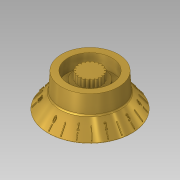
# Autodesk Inventor part: Knob
Saved by Autodesk Inventor 2016 (Build 200138000, 138)
## iProperties
Created: 2018-09-08
Part Number: Knob
Material: Generic
Document SubType Name: Modeling
Designer: Pedro Mendonça
Density: 1 g/cm^3
Appearance: Gold - Metal(1)
Author: Pedro Mendonça
Autodesk Inventor part; units mm, degrees
ref_plane "YZ Plane" through (0, 0, 0) normal (1, 0, 0) x (0, 1, 0)
ref_plane "XZ Plane" through (0, 0, 0) normal (0, 1, 0) x (-1, 0, 0)
sketch "Sketch1" plane through (0, 0, 0) normal (1, 0, 0) x (0, 1, 0)
  line L0 (0, 0) -> (0, 12.45)
  line L1 (0, 12.45) -> (8.7, 12.45)
  line L2 (8.7, 12.45) -> (9.2, 4.8665)
  line L3 (0, 0) -> (13.15, 0)
  line L4 (13.15, 0) -> (9.2, 4.8665)
  line L5 (0, -2.49) -> (0, 14.94) projected
  dimension "d5" = 12.45
  dimension "d6" = 8.7
  dimension "d7" = 7.6
  dimension "d8" = 13.15
  dimension "d10" = 9.2
  constraints: 10 end point, 1 horizontal, 1 perpendicular, 1 vertical
  measures "d5" distance of L0.start L0.end
  measures "d6" distance of L0.end L1.end
  measures "d7" distance of L1.end L2.end
  measures "d8" distance of L0.start L3.end
  measures "d10" distance from line of L2.end L0
revolve "Revolution1" add sketch "Sketch1" angle 360 about axis through (0, 0, -10) along (0, 0, 1)
sketch "Sketch2" plane through (0, 0, 0) normal (1, 0, 0) x (0, 1, 0)
  line L0 (-11.15, 0) -> (-7.2104, 4.8749)
  line L1 (-7.2173, 4.8665) -> (-6.8225, 10.8535)
  line L2 (-6.8225, 10.8535) -> (-4.8225, 10.8535)
  line L3 (-4.8225, 10.8535) -> (-4.8225, 0)
  line L4 (-11.15, 0) -> (-4.8225, 0)
  line L5 (-13.15, 0) -> (13.15, 0) projected
  line L6 (-11.15, 0) -> (-7.2173, 4.8665)
  line L7 (-6.8225, 10.8535) -> (-4.8225, 10.8535)
  line L8 (-4.8225, 0) -> (-11.15, 0)
  line L9 (0, -2.49) -> (0, 14.94) projected
  point P0 (0, 0)
  dimension "d14" = 6
  dimension "d15" = 2
  constraints: 16 end point, 2 horizontal, 2 parallel, 1 collinear
  measures "d14" distance of L1.start L1.end
  measures "d15" distance of L1.end L2.end
revolve "Revolution2" cut sketch "Sketch2" angle 360 about axis through (0, 0, -10) along (0, 0, 1)
sketch "Sketch3" plane through (0, 0, 0) normal (0, 0, -1) x (-1, 0, 0)
  circle A0 centre (0, 0) radius 3.125
  dimension "d17" = 6.25
  constraints: 1 centre point, 1 coincident
  measures "d17" diameter of A0
extrude "Extrusion1" cut sketch "Sketch3" against normal blind 8
sketch "Sketch4" plane through (0, 0, 0) normal (0, 0, -1) x (-1, 0, 0)
  circle A0 centre (0, 0) radius 3.125 projected
  circle A1 centre (0, -3.125) radius 0.485
  circle A2 centre (0.9657, -2.9721) radius 0.485
  circle A3 centre (1.8368, -2.5282) radius 0.485
  circle A4 centre (2.5282, -1.8368) radius 0.485
  circle A5 centre (2.9721, -0.9657) radius 0.485
  circle A6 centre (3.125, 0) radius 0.485
  circle A7 centre (2.9721, 0.9657) radius 0.485
  circle A8 centre (2.5282, 1.8368) radius 0.485
  circle A9 centre (1.8368, 2.5282) radius 0.485
  circle A10 centre (0.9657, 2.9721) radius 0.485
  circle A11 centre (0, 3.125) radius 0.485
  circle A12 centre (-0.9657, 2.9721) radius 0.485
  circle A13 centre (-1.8368, 2.5282) radius 0.485
  circle A14 centre (-2.5282, 1.8368) radius 0.485
  circle A15 centre (-2.9721, 0.9657) radius 0.485
  circle A16 centre (-3.125, 0) radius 0.485
  circle A17 centre (-2.9721, -0.9657) radius 0.485
  circle A18 centre (-2.5282, -1.8368) radius 0.485
  circle A19 centre (-1.8368, -2.5282) radius 0.485
  circle A20 centre (-0.9657, -2.9721) radius 0.485
  dimension "d20" = 0.97
  dimension "d23" = 360
  constraints: 20 centre point, 1 vertical alignment, 42 other
  measures "d20" diameter of A1
extrude "Extrusion2" cut sketch "Sketch4" against normal blind 8 contours A0 A6 | A0 A6 | A7 A0 | A0 A7 | A5 A0 | A0 A5 | A8 A0 | A0 A8 | A4 A0 | A0 A4 | A9 A0 | A0 A9 | A3 A0 | A0 A3 | A10 A0 | A0 A10 | A2 A0 | A0 A2 | A11 A0 | A0 A11 | A1 A0 | A0 A1 | A12 A0 | A0 A12 | A20 A0 | A0 A20 | A13 A0 | A0 A13 | A19 A0 | A0 A19 | A14 A0 | A0 A14 | A18 A0 | A0 A18 | A15 A0 | A0 A15 | A17 A0 | A0 A17 | A16 A0 | A0 A16
fillet "Fillet1" radius 1 1 edges at (0, -9.2, 4.8665)
fillet "Fillet3" radius 0.1 1 edges at (0, -13.15, 0)
sketch "Sketch7" plane through (0, 0, 12.45) normal (0, 0, 1) x (1, 0, 0)
  circle A0 centre (0, 0) radius 10
  dimension "d95" = 20
  constraints: 1 centre point, 1 coincident
  measures "d95" diameter of A0
extrude "Extrusion4" cut sketch "Sketch7" against normal blind 2
sketch "Sketch8" plane through (0, 0, 0) normal (0, 0, -1) x (-1, 0, 0)
  circle A0 centre (0, 0) radius 4.8225
  constraints: 1 centre point, 1 coincident
extrude "Extrusion5" cut sketch "Sketch8" against normal blind 2.5
sketch "Sketch9" plane through (0, 0, 10.45) normal (0, 0, 1) x (1, 0, 0)
  circle A0 centre (0, 0) radius 4.8225 projected
  arc A1 (-1.4235, 2.7819) -> (-2.2059, 2.2135) centre (-1.8368, 2.5282) ccw projected
  arc A2 (-0.4942, 3.0857) -> (-1.4139, 2.7868) centre (-0.9657, 2.9721) ccw projected
  arc A3 (0.4835, 3.0874) -> (-0.4835, 3.0874) centre (0, 3.125) ccw projected
  arc A4 (1.4139, 2.7868) -> (0.4942, 3.0857) centre (0.9657, 2.9721) ccw projected
  arc A5 (2.2059, 2.2135) -> (1.4235, 2.7819) centre (1.8368, 2.5282) ccw projected
  arc A6 (2.7819, 1.4235) -> (2.2135, 2.2059) centre (2.5282, 1.8368) ccw projected
  arc A7 (3.0857, 0.4942) -> (2.7868, 1.4139) centre (2.9721, 0.9657) ccw projected
  arc A8 (3.0874, -0.4835) -> (3.0874, 0.4835) centre (3.125, 0) ccw projected
  arc A9 (2.7868, -1.4139) -> (3.0857, -0.4942) centre (2.9721, -0.9657) ccw projected
  arc A10 (2.2135, -2.2059) -> (2.7819, -1.4235) centre (2.5282, -1.8368) ccw projected
  arc A11 (1.4235, -2.7819) -> (2.2059, -2.2135) centre (1.8368, -2.5282) ccw projected
  arc A12 (0.4942, -3.0857) -> (1.4139, -2.7868) centre (0.9657, -2.9721) ccw projected
  arc A13 (-0.4835, -3.0874) -> (0.4835, -3.0874) centre (0, -3.125) ccw projected
  arc A14 (-1.4139, -2.7868) -> (-0.4942, -3.0857) centre (-0.9657, -2.9721) ccw projected
  arc A15 (-2.2059, -2.2135) -> (-1.4235, -2.7819) centre (-1.8368, -2.5282) ccw projected
  arc A16 (-2.7819, -1.4235) -> (-2.2135, -2.2059) centre (-2.5282, -1.8368) ccw projected
  arc A17 (-3.0857, -0.4942) -> (-2.7868, -1.4139) centre (-2.9721, -0.9657) ccw projected
  arc A18 (-3.0874, 0.4835) -> (-3.0874, -0.4835) centre (-3.125, 0) ccw projected
  arc A19 (-2.7868, 1.4139) -> (-3.0857, 0.4942) centre (-2.9721, 0.9657) ccw projected
  arc A20 (-2.2135, 2.2059) -> (-2.7819, 1.4235) centre (-2.5282, 1.8368) ccw projected
  arc A21 (3.0857, -0.4942) -> (3.0874, -0.4835) centre (0, 0) ccw
  arc A22 (3.0874, 0.4835) -> (3.0857, 0.4942) centre (0, 0) ccw
  arc A23 (2.7868, 1.4139) -> (2.7819, 1.4235) centre (0, 0) ccw
  arc A24 (2.2135, 2.2059) -> (2.2059, 2.2135) centre (0, 0) ccw
  arc A25 (1.4235, 2.7819) -> (1.4139, 2.7868) centre (0, 0) ccw
  arc A26 (0.4942, 3.0857) -> (0.4835, 3.0874) centre (0, 0) ccw
  arc A27 (-0.4835, 3.0874) -> (-0.4942, 3.0857) centre (0, 0) ccw
  arc A28 (-1.4139, 2.7868) -> (-1.4235, 2.7819) centre (0, 0) ccw
  arc A29 (-2.2059, 2.2135) -> (-2.2135, 2.2059) centre (0, 0) ccw
  arc A30 (-2.7819, 1.4235) -> (-2.7868, 1.4139) centre (0, 0) ccw
  arc A31 (-3.0857, 0.4942) -> (-3.0874, 0.4835) centre (0, 0) ccw
  arc A32 (-3.0874, -0.4835) -> (-3.0857, -0.4942) centre (0, 0) ccw
  arc A33 (-2.7868, -1.4139) -> (-2.7819, -1.4235) centre (0, 0) ccw
  arc A34 (-2.2135, -2.2059) -> (-2.2059, -2.2135) centre (0, 0) ccw
  arc A35 (-1.4235, -2.7819) -> (-1.4139, -2.7868) centre (0, 0) ccw
  arc A36 (-0.4942, -3.0857) -> (-0.4835, -3.0874) centre (0, 0) ccw
  arc A37 (0.4835, -3.0874) -> (0.4942, -3.0857) centre (0, 0) ccw
  arc A38 (1.4139, -2.7868) -> (1.4235, -2.7819) centre (0, 0) ccw
  arc A39 (2.2059, -2.2135) -> (2.2135, -2.2059) centre (0, 0) ccw
  arc A40 (2.7819, -1.4235) -> (2.7868, -1.4139) centre (0, 0) ccw
  constraints: 80 point on circle, 20 centre point, 1 coincident
extrude "Extrusion6" cut sketch "Sketch9" against normal blind 2.3
ref_plane "Work Plane2" through (0, 0, 6.15) normal (0, 0, 1) x (1, 0, 0)
sketch "Sketch11" plane through (0, 0, 6.15) normal (0, 0, 1) x (1, 0, 0)
  circle A0 centre (0, 0) radius 7.75
  circle A1 centre (0, 0) radius 4.8212
  dimension "d106" = 15.5
  constraints: 2 centre point, 2 coincident
  measures "d106" diameter of A0
extrude "Extrusion9" add sketch "Sketch11" against normal blind 1
ref_plane "Work Plane3" through (0, 0, 20) normal (0, 0, 1) x (1, 0, 0)
sketch "Sketch12" plane through (0, 0, 20) normal (0, 0, 1) x (1, 0, 0)
  line L0 (12.8, -0.1) -> (11.8, -0.1)
  line L1 (11.8, -0.1) -> (11.8, 0.1)
  line L2 (11.8, 0.1) -> (12.8, 0.1)
  line L3 (12.8, 0.1) -> (12.8, -0.1)
  line L4 (12.8, -0.1) -> (11.8, 0.1) construction
  line L5 (11.8, -0.1) -> (12.8, 0.1) construction
  line L6 (10.4579, 2.6987) -> (12.3897, 3.2163)
  line L7 (12.3897, 3.2163) -> (12.338, 3.4095)
  line L8 (12.338, 3.4095) -> (10.4061, 2.8918)
  line L9 (10.4061, 2.8918) -> (10.4579, 2.6987)
  line L10 (10.9468, 6.6346) -> (10.0957, 6.1096)
  line L11 (10.0957, 6.1096) -> (9.9907, 6.2798)
  line L12 (9.9907, 6.2798) -> (10.8418, 6.8048)
  line L13 (10.8418, 6.8048) -> (10.9468, 6.6346)
  line L14 (10.9468, 6.6346) -> (9.9907, 6.2798) construction
  line L15 (10.0957, 6.1096) -> (10.8418, 6.8048) construction
  line L16 (7.4841, 7.787) -> (8.8566, 9.2418)
  line L17 (8.8566, 9.2418) -> (8.7112, 9.379)
  line L18 (8.7112, 9.379) -> (7.3387, 7.9243)
  line L19 (7.3387, 7.9243) -> (7.4841, 7.787)
  line L20 (5.834, 11.3936) -> (5.3852, 10.5)
  line L21 (5.3852, 10.5) -> (5.2065, 10.5897)
  line L22 (5.2065, 10.5897) -> (5.6553, 11.4834)
  line L23 (5.6553, 11.4834) -> (5.834, 11.3936)
  line L24 (5.834, 11.3936) -> (5.2065, 10.5897) construction
  line L25 (5.3852, 10.5) -> (5.6553, 11.4834) construction
  line L26 (2.2819, 10.5567) -> (2.6863, 12.5153)
  line L27 (2.6863, 12.5153) -> (2.4905, 12.5558)
  line L28 (2.4905, 12.5558) -> (2.086, 10.5971)
  line L29 (2.086, 10.5971) -> (2.2819, 10.5567)
  line L30 (-1.016, 12.76) -> (-0.9288, 11.7638)
  line L31 (-0.9288, 11.7638) -> (-1.1281, 11.7464)
  line L32 (-1.1281, 11.7464) -> (-1.2152, 12.7426)
  line L33 (-1.2152, 12.7426) -> (-1.016, 12.76)
  line L34 (-1.016, 12.76) -> (-1.1281, 11.7464) construction
  line L35 (-0.9288, 11.7638) -> (-1.2152, 12.7426) construction
  line L36 (-3.5998, 10.1829) -> (-4.2839, 12.0623)
  line L37 (-4.2839, 12.0623) -> (-4.4718, 11.9939)
  line L38 (-4.4718, 11.9939) -> (-3.7878, 10.1145)
  line L39 (-3.7878, 10.1145) -> (-3.5998, 10.1829)
  line L40 (-7.5634, 10.3269) -> (-6.9663, 9.5248)
  line L41 (-6.9663, 9.5248) -> (-7.1267, 9.4053)
  line L42 (-7.1267, 9.4053) -> (-7.7238, 10.2075)
  line L43 (-7.7238, 10.2075) -> (-7.5634, 10.3269)
  line L44 (-7.5634, 10.3269) -> (-7.1267, 9.4053) construction
  line L45 (-6.9663, 9.5248) -> (-7.7238, 10.2075) construction
  line L46 (-8.4097, 6.777) -> (-9.9785, 8.0175)
  line L47 (-9.9785, 8.0175) -> (-10.1025, 7.8606)
  line L48 (-10.1025, 7.8606) -> (-8.5337, 6.6201)
  line L49 (-8.5337, 6.6201) -> (-8.4097, 6.777)
  line L50 (-11.8587, 4.8188) -> (-10.9294, 4.4496)
  line L51 (-10.9294, 4.4496) -> (-11.0032, 4.2637)
  line L52 (-11.0032, 4.2637) -> (-11.9326, 4.6329)
  line L53 (-11.9326, 4.6329) -> (-11.8587, 4.8188)
  line L54 (-11.8587, 4.8188) -> (-11.0032, 4.2637) construction
  line L55 (-10.9294, 4.4496) -> (-11.9326, 4.6329) construction
  line L56 (-10.7154, 1.3531) -> (-12.7018, 1.5853)
  line L57 (-12.7018, 1.5853) -> (-12.7251, 1.3867)
  line L58 (-12.7251, 1.3867) -> (-10.7386, 1.1545)
  line L59 (-10.7386, 1.1545) -> (-10.7154, 1.3531)
  line L60 (-12.6229, -2.1242) -> (-11.6381, -1.9506)
  line L61 (-11.6381, -1.9506) -> (-11.6034, -2.1475)
  line L62 (-11.6034, -2.1475) -> (-12.5882, -2.3212)
  line L63 (-12.5882, -2.3212) -> (-12.6229, -2.1242)
  line L64 (-12.6229, -2.1242) -> (-11.6034, -2.1475) construction
  line L65 (-11.6381, -1.9506) -> (-12.5882, -2.3212) construction
  line L66 (-9.8304, -4.4736) -> (-11.643, -5.3189)
  line L67 (-11.643, -5.3189) -> (-11.5585, -5.5001)
  line L68 (-11.5585, -5.5001) -> (-9.7459, -4.6549)
  line L69 (-9.7459, -4.6549) -> (-9.8304, -4.4736)
  line L70 (-9.6284, -8.4347) -> (-8.8814, -7.7699)
  line L71 (-8.8814, -7.7699) -> (-8.7484, -7.9193)
  line L72 (-8.7484, -7.9193) -> (-9.4954, -8.5841)
  line L73 (-9.4954, -8.5841) -> (-9.6284, -8.4347)
  line L74 (-9.6284, -8.4347) -> (-8.7484, -7.9193) construction
  line L75 (-8.8814, -7.7699) -> (-9.4954, -8.5841) construction
  line L76 (-6.0182, -8.9683) -> (-7.1173, -10.6393)
  line L77 (-7.1173, -10.6393) -> (-6.9502, -10.7492)
  line L78 (-6.9502, -10.7492) -> (-5.8511, -9.0782)
  line L79 (-5.8511, -9.0782) -> (-6.0182, -8.9683)
  line L80 (-3.7669, -12.2336) -> (-3.4801, -11.2756)
  line L81 (-3.4801, -11.2756) -> (-3.2885, -11.333)
  line L82 (-3.2885, -11.333) -> (-3.5753, -12.2909)
  line L83 (-3.5753, -12.2909) -> (-3.7669, -12.2336)
  line L84 (-3.7669, -12.2336) -> (-3.2885, -11.333) construction
  line L85 (-3.4801, -11.2756) -> (-3.5753, -12.2909) construction
  line L86 (-0.4141, -10.7925) -> (-0.4722, -12.7917)
  line L87 (-0.4722, -12.7917) -> (-0.2723, -12.7975)
  line L88 (-0.2723, -12.7975) -> (-0.2142, -10.7983)
  line L89 (-0.2142, -10.7983) -> (-0.4141, -10.7925)
  line L90 (3.2163, -12.3897) -> (2.9575, -11.4238)
  line L91 (2.9575, -11.4238) -> (3.1507, -11.372)
  line L92 (3.1507, -11.372) -> (3.4095, -12.338)
  line L93 (3.4095, -12.338) -> (3.2163, -12.3897)
  line L94 (3.2163, -12.3897) -> (3.1507, -11.372) construction
  line L95 (2.9575, -11.4238) -> (3.4095, -12.338) construction
  line L96 (5.3134, -9.4031) -> (6.3134, -11.1351)
  line L97 (6.3134, -11.1351) -> (6.4866, -11.0351)
  line L98 (6.4866, -11.0351) -> (5.4866, -9.3031)
  line L99 (5.4866, -9.3031) -> (5.3134, -9.4031)
  line L100 (8.2731, -8.4146) -> (8.4146, -8.2731)
  line L101 (8.4146, -8.2731) -> (9.1217, -8.9803)
  line L102 (8.9803, -9.1217) -> (8.2731, -8.4146)
  line L103 (8.9803, -9.1217) -> (8.4146, -8.2731) construction
  line L104 (8.2731, -8.4146) -> (9.1217, -8.9803) construction
  line L105 (9.1217, -8.9803) -> (8.9803, -9.1217)
  line L106 (10.4323, -0.3696) -> (10.4323, 0.5179) construction
  line L107 (10.4323, 0.5179) -> (11.6764, 0.5179) construction
  line L108 (11.6764, 0.5179) -> (11.6764, -0.3696) construction
  line L109 (11.6764, -0.3696) -> (10.4323, -0.3696) construction
  line L110 (9.0791, 5.1516) -> (8.6141, 5.9075) construction
  line L111 (8.6141, 5.9075) -> (9.6738, 6.5594) construction
  line L112 (9.6738, 6.5594) -> (10.1388, 5.8035) construction
  line L113 (10.1388, 5.8035) -> (9.0791, 5.1516) construction
  line L114 (4.9856, 9.1713) -> (4.1914, 9.5673) construction
  line L115 (4.1914, 9.5673) -> (4.7465, 10.6807) construction
  line L116 (4.7465, 10.6807) -> (5.5407, 10.2847) construction
  line L117 (5.5407, 10.2847) -> (4.9856, 9.1713) construction
  line L118 (-0.6698, 11.663) -> (-0.5592, 10.4238) construction
  line L119 (-0.5592, 10.4238) -> (-1.4432, 10.3449) construction
  line L120 (-1.4432, 10.3449) -> (-1.5538, 11.5842) construction
  line L121 (-1.5538, 11.5842) -> (-0.6698, 11.663) construction
  line L122 (-5.9233, 8.5956) -> (-6.6358, 8.0664) construction
  line L123 (-6.6358, 8.0664) -> (-7.3775, 9.0653) construction
  line L124 (-7.3775, 9.0653) -> (-6.6651, 9.5944) construction
  line L125 (-6.6651, 9.5944) -> (-5.9233, 8.5956) construction
  line L126 (-10.7041, 4.6794) -> (-9.549, 4.2174) construction
  line L127 (-9.549, 4.2174) -> (-9.8786, 3.3934) construction
  line L128 (-9.8786, 3.3934) -> (-11.0337, 3.8554) construction
  line L129 (-11.0337, 3.8554) -> (-10.7041, 4.6794) construction
  line L130 (-11.5603, -1.6838) -> (-10.3354, -1.4656) construction
  line L131 (-10.3354, -1.4656) -> (-10.1798, -2.3393) construction
  line L132 (-10.1798, -2.3393) -> (-11.4047, -2.5575) construction
  line L133 (-11.4047, -2.5575) -> (-11.5603, -1.6838) construction
  line L134 (-8.9639, -7.4916) -> (-8.035, -6.6639) construction
  line L135 (-8.035, -6.6639) -> (-7.4446, -7.3265) construction
  line L136 (-7.4446, -7.3265) -> (-8.3735, -8.1542) construction
  line L137 (-8.3735, -8.1542) -> (-8.9639, -7.4916) construction
  line L138 (-3.7669, -11.1351) -> (-3.363, -9.8771) construction
  line L139 (-3.363, -9.8771) -> (-2.5697, -10.1318) construction
  line L140 (-2.5697, -10.1318) -> (-2.9736, -11.3898) construction
  line L141 (-2.9736, -11.3898) -> (-3.7669, -11.1351) construction
  line L142 (2.5884, -11.3898) -> (2.2851, -10.1824) construction
  line L143 (2.2851, -10.1824) -> (3.4005, -9.9022) construction
  line L144 (3.4005, -9.9022) -> (3.7038, -11.1097) construction
  line L145 (3.7038, -11.1097) -> (2.5884, -11.3898) construction
  line L146 (7.6666, -8.7681) -> (6.8232, -7.9451) construction
  line L147 (6.8232, -7.9451) -> (8.3823, -6.3474) construction
  line L148 (8.3823, -6.3474) -> (9.2258, -7.1704) construction
  line L149 (9.2258, -7.1704) -> (7.6666, -8.7681) construction
  spline S0 degree 2 poles (10.9525, 0.3257) (11.2216, 0.3257) (11.4736, 0.1693) (11.4736, 0.0064) knots 0 0 0 1 2 2 2
  spline S1 degree 2 poles (11.4736, 0.0064) (11.4736, -0.1589) (11.2167, -0.3137) (10.9533, -0.3137) knots 0 0 0 1 2 2 2
  spline S2 degree 2 poles (10.9533, -0.3137) (10.6827, -0.3137) (10.4323, -0.1573) (10.4323, 0.0064) knots 0 0 0 1 2 2 2
  spline S3 degree 2 poles (10.4323, 0.0064) (10.4323, 0.1709) (10.6916, 0.3257) (10.9525, 0.3257) knots 0 0 0 1 2 2 2
  spline S4 degree 2 poles (11.2572, 0.1539) (11.2078, 0.1734) (11.0555, 0.1896) (10.9525, 0.1896) knots 0 0 0 1 2 2 2
  spline S5 degree 2 poles (10.9525, 0.1896) (10.8496, 0.1896) (10.6981, 0.1734) (10.647, 0.1531) knots 0 0 0 1 2 2 2
  spline S6 degree 2 poles (10.647, 0.1531) (10.596, 0.1328) (10.5433, 0.0623) (10.5433, 0.0064) knots 0 0 0 1 2 2 2
  spline S7 degree 2 poles (10.5433, 0.0064) (10.5433, -0.0495) (10.596, -0.1216) (10.6486, -0.1427) knots 0 0 0 1 2 2 2
  spline S8 degree 2 poles (10.6486, -0.1427) (10.6997, -0.1629) (10.8553, -0.1775) (10.9533, -0.1775) knots 0 0 0 1 2 2 2
  spline S9 degree 2 poles (10.9533, -0.1775) (11.0587, -0.1775) (11.1997, -0.1646) (11.2548, -0.1435) knots 0 0 0 1 2 2 2
  spline S10 degree 2 poles (11.2548, -0.1435) (11.3067, -0.124) (11.3626, -0.0519) (11.3626, 0.0064) knots 0 0 0 1 2 2 2
  spline S11 degree 2 poles (11.3626, 0.0064) (11.3626, 0.0615) (11.3099, 0.1337) (11.2572, 0.1539) knots 0 0 0 1 2 2 2
  line L150 (9.5986, 6.2218) -> (9.8542, 5.8063)
  line L151 (9.8542, 5.8063) -> (9.7672, 5.7528)
  line L152 (9.7672, 5.7528) -> (9.6721, 5.9074)
  line L153 (9.6721, 5.9074) -> (9.1013, 5.5563)
  line L154 (9.1013, 5.5563) -> (9.1964, 5.4017)
  line L155 (9.1964, 5.4017) -> (9.1184, 5.3537)
  spline S12 degree 2 poles (9.1184, 5.3537) (9.0645, 5.4413) (8.9638, 5.4936) (8.8914, 5.4567) knots 0 0 0 1 2 2 2
  line L156 (8.8914, 5.4567) -> (8.8371, 5.545)
  line L157 (8.8371, 5.545) -> (9.6046, 6.0172)
  line L158 (9.6046, 6.0172) -> (9.5116, 6.1683)
  line L159 (9.5116, 6.1683) -> (9.5986, 6.2218)
  line L160 (4.824, 10.3928) -> (5.3759, 10.1176)
  line L161 (5.3759, 10.1176) -> (5.3127, 9.9907)
  spline S13 degree 2 poles (5.3127, 9.9907) (5.2254, 9.9645) (5.0678, 9.9136) (4.9892, 9.8831) knots 0 0 0 1 2 2 2
  spline S14 degree 2 poles (4.9892, 9.8831) (4.8309, 9.8216) (4.6889, 9.724) (4.6531, 9.6522) knots 0 0 0 1 2 2 2
  spline S15 degree 2 poles (4.6531, 9.6522) (4.6343, 9.6145) (4.6293, 9.5463) (4.6413, 9.5177) knots 0 0 0 1 2 2 2
  spline S16 degree 2 poles (4.6413, 9.5177) (4.6533, 9.4891) (4.6994, 9.4435) (4.7327, 9.4269) knots 0 0 0 1 2 2 2
  spline S17 degree 2 poles (4.7327, 9.4269) (4.7646, 9.411) (4.8379, 9.3944) (4.8737, 9.3919) knots 0 0 0 1 2 2 2
  spline S18 degree 2 poles (4.8737, 9.3919) (4.9042, 9.3894) (4.9658, 9.3949) (4.9854, 9.3978) knots 0 0 0 1 2 2 2
  line L162 (4.9854, 9.3978) -> (4.9919, 9.3945)
  line L163 (4.9919, 9.3945) -> (4.9282, 9.2669)
  spline S19 degree 2 poles (4.9282, 9.2669) (4.8822, 9.2672) (4.7318, 9.2979) (4.6723, 9.3275) knots 0 0 0 1 2 2 2
  spline S20 degree 2 poles (4.6723, 9.3275) (4.5468, 9.3901) (4.4716, 9.5933) (4.528, 9.7064) knots 0 0 0 1 2 2 2
  spline S21 degree 2 poles (4.528, 9.7064) (4.5544, 9.7594) (4.6232, 9.8355) (4.6637, 9.8624) knots 0 0 0 1 2 2 2
  spline S22 degree 2 poles (4.6637, 9.8624) (4.705, 9.8907) (4.8064, 9.9361) (4.8597, 9.9558) knots 0 0 0 1 2 2 2
  spline S23 degree 2 poles (4.8597, 9.9558) (4.947, 9.9892) (5.1513, 10.0521) (5.2118, 10.07) knots 0 0 0 1 2 2 2
  line L164 (5.2118, 10.07) -> (4.7723, 10.2891)
  line L165 (4.7723, 10.2891) -> (4.824, 10.3928)
  spline S24 degree 2 poles (-0.911, 10.5088) (-0.8747, 10.512) (-0.8044, 10.5362) (-0.7709, 10.553) knots 0 0 0 1 2 2 2
  spline S25 degree 2 poles (-0.7709, 10.553) (-0.7399, 10.5696) (-0.6948, 10.6029) (-0.6774, 10.6175) knots 0 0 0 1 2 2 2
  line L166 (-0.6774, 10.6175) -> (-0.6693, 10.6182)
  line L167 (-0.6693, 10.6182) -> (-0.6567, 10.477)
  spline S26 degree 2 poles (-0.6567, 10.477) (-0.6982, 10.4497) (-0.8442, 10.3984) (-0.9112, 10.3924) knots 0 0 0 1 2 2 2
  spline S27 degree 2 poles (-0.9112, 10.3924) (-0.979, 10.3864) (-1.0823, 10.4048) (-1.1261, 10.4302) knots 0 0 0 1 2 2 2
  spline S28 degree 2 poles (-1.1261, 10.4302) (-1.1725, 10.4578) (-1.2258, 10.545) (-1.2313, 10.6063) knots 0 0 0 1 2 2 2
  spline S29 degree 2 poles (-1.2313, 10.6063) (-1.2386, 10.6886) (-1.1416, 10.8226) (-1.0671, 10.8455) knots 0 0 0 1 2 2 2
  line L168 (-1.0671, 10.8455) -> (-1.068, 10.8552)
  spline S30 degree 2 poles (-1.068, 10.8552) (-1.1001, 10.8588) (-1.1745, 10.8815) (-1.2078, 10.9078) knots 0 0 0 1 2 2 2
  spline S31 degree 2 poles (-1.2078, 10.9078) (-1.2409, 10.9333) (-1.2878, 11.0203) (-1.2936, 11.0856) knots 0 0 0 1 2 2 2
  spline S32 degree 2 poles (-1.2936, 11.0856) (-1.2996, 11.1526) (-1.2637, 11.2706) (-1.2256, 11.3179) knots 0 0 0 1 2 2 2
  spline S33 degree 2 poles (-1.2256, 11.3179) (-1.1861, 11.367) (-1.0668, 11.4248) (-0.9885, 11.4318) knots 0 0 0 1 2 2 2
  spline S34 degree 2 poles (-0.9885, 11.4318) (-0.9134, 11.4385) (-0.7633, 11.4153) (-0.711, 11.3947) knots 0 0 0 1 2 2 2
  line L169 (-0.711, 11.3947) -> (-0.6984, 11.2535)
  line L170 (-0.6984, 11.2535) -> (-0.7081, 11.2526)
  spline S35 degree 2 poles (-0.7081, 11.2526) (-0.7528, 11.2795) (-0.8999, 11.3234) (-0.9701, 11.3171) knots 0 0 0 1 2 2 2
  spline S36 degree 2 poles (-0.9701, 11.3171) (-1.0113, 11.3134) (-1.0913, 11.2803) (-1.1161, 11.2479) knots 0 0 0 1 2 2 2
  spline S37 degree 2 poles (-1.1161, 11.2479) (-1.14, 11.2157) (-1.162, 11.1421) (-1.1571, 11.0881) knots 0 0 0 1 2 2 2
  spline S38 degree 2 poles (-1.1571, 11.0881) (-1.1523, 11.034) (-1.1146, 10.9666) (-1.0845, 10.9489) knots 0 0 0 1 2 2 2
  spline S39 degree 2 poles (-1.0845, 10.9489) (-1.0545, 10.9313) (-0.9764, 10.9228) (-0.9312, 10.9268) knots 0 0 0 1 2 2 2
  line L171 (-0.9312, 10.9268) -> (-0.8747, 10.9318)
  line L172 (-0.8747, 10.9318) -> (-0.8648, 10.8213)
  line L173 (-0.8648, 10.8213) -> (-0.9092, 10.8173)
  spline S40 degree 2 poles (-0.9092, 10.8173) (-0.9988, 10.8093) (-1.1042, 10.7137) (-1.0969, 10.6321) knots 0 0 0 1 2 2 2
  spline S41 degree 2 poles (-1.0969, 10.6321) (-1.0935, 10.5942) (-1.0596, 10.5427) (-1.0348, 10.5287) knots 0 0 0 1 2 2 2
  spline S42 degree 2 poles (-1.0348, 10.5287) (-1.0083, 10.5139) (-0.9457, 10.5057) (-0.911, 10.5088) knots 0 0 0 1 2 2 2
  line L174 (-6.8898, 8.6954) -> (-6.7941, 8.7665)
  line L175 (-6.7941, 8.7665) -> (-6.999, 9.0423)
  line L176 (-6.999, 9.0423) -> (-6.8955, 9.1191)
  line L177 (-6.8955, 9.1191) -> (-6.6907, 8.8433)
  line L178 (-6.6907, 8.8433) -> (-6.3361, 9.1066)
  line L179 (-6.3361, 9.1066) -> (-6.252, 8.9934)
  line L180 (-6.252, 8.9934) -> (-6.3039, 8.3129)
  line L181 (-6.3039, 8.3129) -> (-6.4028, 8.2395)
  line L182 (-6.4028, 8.2395) -> (-6.7299, 8.6799)
  line L183 (-6.7299, 8.6799) -> (-6.8255, 8.6089)
  line L184 (-6.8255, 8.6089) -> (-6.8898, 8.6954)
  line L185 (-6.6264, 8.7567) -> (-6.3935, 8.4432)
  line L186 (-6.3935, 8.4432) -> (-6.3564, 8.9573)
  line L187 (-6.3564, 8.9573) -> (-6.6264, 8.7567)
  spline S43 degree 2 poles (-10.4347, 3.8402) (-10.5017, 3.867) (-10.5989, 3.9557) (-10.6254, 4.0116) knots 0 0 0 1 2 2 2
  spline S44 degree 2 poles (-10.6254, 4.0116) (-10.6519, 4.0676) (-10.6541, 4.2038) (-10.6252, 4.276) knots 0 0 0 1 2 2 2
  spline S45 degree 2 poles (-10.6252, 4.276) (-10.5987, 4.3422) (-10.5176, 4.4599) (-10.4753, 4.498) knots 0 0 0 1 2 2 2
  line L188 (-10.4753, 4.498) -> (-10.3437, 4.4453)
  line L189 (-10.3437, 4.4453) -> (-10.3473, 4.4363)
  spline S46 degree 2 poles (-10.3473, 4.4363) (-10.3635, 4.4262) (-10.412, 4.3836) (-10.437, 4.3561) knots 0 0 0 1 2 2 2
  spline S47 degree 2 poles (-10.437, 4.3561) (-10.4645, 4.3243) (-10.5032, 4.2691) (-10.5185, 4.2307) knots 0 0 0 1 2 2 2
  spline S48 degree 2 poles (-10.5185, 4.2307) (-10.5336, 4.1931) (-10.5348, 4.1116) (-10.5157, 4.0742) knots 0 0 0 1 2 2 2
  spline S49 degree 2 poles (-10.5157, 4.0742) (-10.4972, 4.0398) (-10.4331, 3.9862) (-10.3834, 3.9663) knots 0 0 0 1 2 2 2
  spline S50 degree 2 poles (-10.3834, 3.9663) (-10.3337, 3.9465) (-10.2597, 3.9483) (-10.2284, 3.9654) knots 0 0 0 1 2 2 2
  spline S51 degree 2 poles (-10.2284, 3.9654) (-10.1945, 3.9824) (-10.1437, 4.0529) (-10.1247, 4.1003) knots 0 0 0 1 2 2 2
  spline S52 degree 2 poles (-10.1247, 4.1003) (-10.1043, 4.1514) (-10.0794, 4.2593) (-10.0739, 4.2929) knots 0 0 0 1 2 2 2
  line L190 (-10.0739, 4.2929) -> (-9.5953, 4.1015)
  line L191 (-9.5953, 4.1015) -> (-9.7991, 3.5921)
  line L192 (-9.7991, 3.5921) -> (-9.9082, 3.6357)
  line L193 (-9.9082, 3.6357) -> (-9.7523, 4.0255)
  line L194 (-9.7523, 4.0255) -> (-9.9998, 4.1245)
  spline S53 degree 2 poles (-9.9998, 4.1245) (-10.0058, 4.1007) (-10.021, 4.0562) (-10.0283, 4.0381) knots 0 0 0 1 2 2 2
  spline S54 degree 2 poles (-10.0283, 4.0381) (-10.0568, 3.9667) (-10.1196, 3.8774) (-10.1723, 3.8461) knots 0 0 0 1 2 2 2
  spline S55 degree 2 poles (-10.1723, 3.8461) (-10.2252, 3.8141) (-10.3504, 3.8065) (-10.4347, 3.8402) knots 0 0 0 1 2 2 2
  spline S56 degree 2 poles (-10.8955, -2.2815) (-10.9713, -2.295) (-11.1087, -2.2676) (-11.1593, -2.233) knots 0 0 0 1 2 2 2
  spline S57 degree 2 poles (-11.1593, -2.233) (-11.2126, -2.1972) (-11.2793, -2.0955) (-11.2911, -2.0293) knots 0 0 0 1 2 2 2
  spline S58 degree 2 poles (-11.2911, -2.0293) (-11.3029, -1.9631) (-11.2777, -1.8458) (-11.2404, -1.7964) knots 0 0 0 1 2 2 2
  spline S59 degree 2 poles (-11.2404, -1.7964) (-11.196, -1.7358) (-11.0268, -1.6464) (-10.8959, -1.6231) knots 0 0 0 1 2 2 2
  spline S60 degree 2 poles (-10.8959, -1.6231) (-10.7675, -1.6002) (-10.5515, -1.616) (-10.4651, -1.6574) knots 0 0 0 1 2 2 2
  spline S61 degree 2 poles (-10.4651, -1.6574) (-10.3805, -1.6975) (-10.2666, -1.8518) (-10.2469, -1.9627) knots 0 0 0 1 2 2 2
  spline S62 degree 2 poles (-10.2469, -1.9627) (-10.2411, -1.9954) (-10.2372, -2.0539) (-10.2406, -2.0768) knots 0 0 0 1 2 2 2
  line L195 (-10.2406, -2.0768) -> (-10.3674, -2.0994)
  line L196 (-10.3674, -2.0994) -> (-10.3684, -2.0938)
  spline S63 degree 2 poles (-10.3684, -2.0938) (-10.3621, -2.0737) (-10.3573, -2.0037) (-10.3641, -1.9654) knots 0 0 0 1 2 2 2
  spline S64 degree 2 poles (-10.3641, -1.9654) (-10.386, -1.8426) (-10.5788, -1.7213) (-10.7441, -1.736) knots 0 0 0 1 2 2 2
  spline S65 degree 2 poles (-10.7441, -1.736) (-10.703, -1.7772) (-10.6495, -1.8697) (-10.639, -1.9288) knots 0 0 0 1 2 2 2
  spline S66 degree 2 poles (-10.639, -1.9288) (-10.6287, -1.9862) (-10.6365, -2.0765) (-10.6632, -2.1298) knots 0 0 0 1 2 2 2
  spline S67 degree 2 poles (-10.6632, -2.1298) (-10.6943, -2.1913) (-10.8109, -2.2664) (-10.8955, -2.2815) knots 0 0 0 1 2 2 2
  spline S68 degree 2 poles (-10.925, -2.1485) (-10.8643, -2.1377) (-10.7878, -2.0911) (-10.7654, -2.0509) knots 0 0 0 1 2 2 2
  spline S69 degree 2 poles (-10.7654, -2.0509) (-10.7493, -2.0209) (-10.7474, -1.953) (-10.7535, -1.9187) knots 0 0 0 1 2 2 2
  spline S70 degree 2 poles (-10.7535, -1.9187) (-10.7618, -1.8725) (-10.8052, -1.7905) (-10.839, -1.7529) knots 0 0 0 1 2 2 2
  spline S71 degree 2 poles (-10.839, -1.7529) (-10.8535, -1.7546) (-10.881, -1.7579) (-10.9017, -1.7616) knots 0 0 0 1 2 2 2
  spline S72 degree 2 poles (-10.9017, -1.7616) (-11.0038, -1.7798) (-11.122, -1.842) (-11.1493, -1.8781) knots 0 0 0 1 2 2 2
  spline S73 degree 2 poles (-11.1493, -1.8781) (-11.1754, -1.9116) (-11.1894, -1.9766) (-11.1832, -2.0109) knots 0 0 0 1 2 2 2
  spline S74 degree 2 poles (-11.1832, -2.0109) (-11.169, -2.0907) (-11.0383, -2.1686) (-10.925, -2.1485) knots 0 0 0 1 2 2 2
  line L197 (-7.6806, -7.287) -> (-8.6032, -7.5294)
  line L198 (-8.6032, -7.5294) -> (-8.6981, -7.4229)
  line L199 (-8.6981, -7.4229) -> (-7.7351, -7.1771)
  line L200 (-7.7351, -7.1771) -> (-8.0785, -6.7917)
  line L201 (-8.0785, -6.7917) -> (-7.9908, -6.7135)
  line L202 (-7.9908, -6.7135) -> (-7.5687, -7.1873)
  line L203 (-7.5687, -7.1873) -> (-7.6806, -7.287)
  spline S75 degree 2 poles (-3.3253, -10.9871) (-3.3963, -10.9643) (-3.4992, -10.8845) (-3.5274, -10.832) knots 0 0 0 1 2 2 2
  spline S76 degree 2 poles (-3.5274, -10.832) (-3.5552, -10.7805) (-3.5631, -10.6622) (-3.544, -10.6028) knots 0 0 0 1 2 2 2
  spline S77 degree 2 poles (-3.544, -10.6028) (-3.5193, -10.5256) (-3.3951, -10.4225) (-3.304, -10.4092) knots 0 0 0 1 2 2 2
  line L204 (-3.304, -10.4092) -> (-3.3028, -10.4054)
  spline S78 degree 2 poles (-3.3028, -10.4054) (-3.3599, -10.3419) (-3.3965, -10.2229) (-3.3733, -10.1504) knots 0 0 0 1 2 2 2
  spline S79 degree 2 poles (-3.3733, -10.1504) (-3.3388, -10.0431) (-3.1307, -9.9516) (-3.0057, -9.9918) knots 0 0 0 1 2 2 2
  spline S80 degree 2 poles (-3.0057, -9.9918) (-2.8761, -10.0334) (-2.7631, -10.2195) (-2.7972, -10.3259) knots 0 0 0 1 2 2 2
  spline S81 degree 2 poles (-2.7972, -10.3259) (-2.8178, -10.39) (-2.9328, -10.4909) (-3.0144, -10.5039) knots 0 0 0 1 2 2 2
  line L205 (-3.0144, -10.5039) -> (-3.0156, -10.5078)
  spline S82 degree 2 poles (-3.0156, -10.5078) (-2.9447, -10.5731) (-2.8947, -10.7117) (-2.923, -10.7997) knots 0 0 0 1 2 2 2
  spline S83 degree 2 poles (-2.923, -10.7997) (-2.9621, -10.9216) (-3.1926, -11.0297) (-3.3253, -10.9871) knots 0 0 0 1 2 2 2
  spline S84 degree 2 poles (-3.0581, -10.7699) (-3.0393, -10.7112) (-3.0633, -10.6269) (-3.1174, -10.5704) knots 0 0 0 1 2 2 2
  spline S85 degree 2 poles (-3.1174, -10.5704) (-3.1351, -10.5511) (-3.1985, -10.4993) (-3.238, -10.4661) knots 0 0 0 1 2 2 2
  spline S86 degree 2 poles (-3.238, -10.4661) (-3.3016, -10.484) (-3.3912, -10.5693) (-3.4122, -10.6349) knots 0 0 0 1 2 2 2
  spline S87 degree 2 poles (-3.4122, -10.6349) (-3.44, -10.7213) (-3.372, -10.8674) (-3.2933, -10.8927) knots 0 0 0 1 2 2 2
  spline S88 degree 2 poles (-3.2933, -10.8927) (-3.213, -10.9184) (-3.0848, -10.8532) (-3.0581, -10.7699) knots 0 0 0 1 2 2 2
  spline S89 degree 2 poles (-2.9227, -10.2874) (-2.9022, -10.2233) (-2.9603, -10.1102) (-3.0367, -10.0856) knots 0 0 0 1 2 2 2
  spline S90 degree 2 poles (-3.0367, -10.0856) (-3.1062, -10.0633) (-3.2194, -10.1112) (-3.2405, -10.1768) knots 0 0 0 1 2 2 2
  spline S91 degree 2 poles (-3.2405, -10.1768) (-3.2556, -10.2239) (-3.2311, -10.3041) (-3.194, -10.3449) knots 0 0 0 1 2 2 2
  spline S92 degree 2 poles (-3.194, -10.3449) (-3.1782, -10.3619) (-3.1085, -10.426) (-3.0788, -10.4475) knots 0 0 0 1 2 2 2
  spline S93 degree 2 poles (-3.0788, -10.4475) (-3.0097, -10.4229) (-2.9413, -10.3452) (-2.9227, -10.2874) knots 0 0 0 1 2 2 2
  spline S94 degree 2 poles (2.4132, -10.5061) (2.3945, -10.4315) (2.412, -10.295) (2.4432, -10.2396) knots 0 0 0 1 2 2 2
  spline S95 degree 2 poles (2.4432, -10.2396) (2.4724, -10.1863) (2.5775, -10.1089) (2.6372, -10.0939) knots 0 0 0 1 2 2 2
  spline S96 degree 2 poles (2.6372, -10.0939) (2.704, -10.0771) (2.8237, -10.0947) (2.8745, -10.1271) knots 0 0 0 1 2 2 2
  spline S97 degree 2 poles (2.8745, -10.1271) (2.9382, -10.1679) (3.0366, -10.327) (3.07, -10.4598) knots 0 0 0 1 2 2 2
  spline S98 degree 2 poles (3.07, -10.4598) (3.1002, -10.5801) (3.1001, -10.809) (3.0654, -10.8938) knots 0 0 0 1 2 2 2
  spline S99 degree 2 poles (3.0654, -10.8938) (3.0285, -10.9832) (2.8913, -11.1021) (2.7765, -11.1309) knots 0 0 0 1 2 2 2
  spline S100 degree 2 poles (2.7765, -11.1309) (2.7506, -11.1375) (2.6903, -11.1468) (2.6631, -11.1452) knots 0 0 0 1 2 2 2
  line L206 (2.6631, -11.1452) -> (2.6317, -11.0202)
  line L207 (2.6317, -11.0202) -> (2.638, -11.0187)
  spline S101 degree 2 poles (2.638, -11.0187) (2.6569, -11.024) (2.7302, -11.0231) (2.7656, -11.0142) knots 0 0 0 1 2 2 2
  spline S102 degree 2 poles (2.7656, -11.0142) (2.8929, -10.9822) (2.9961, -10.7775) (2.9672, -10.6193) knots 0 0 0 1 2 2 2
  spline S103 degree 2 poles (2.9672, -10.6193) (2.9242, -10.6677) (2.838, -10.7236) (2.7822, -10.7376) knots 0 0 0 1 2 2 2
  spline S104 degree 2 poles (2.7822, -10.7376) (2.7287, -10.7511) (2.634, -10.7498) (2.5807, -10.7273) knots 0 0 0 1 2 2 2
  spline S105 degree 2 poles (2.5807, -10.7273) (2.5188, -10.7002) (2.4347, -10.5918) (2.4132, -10.5061) knots 0 0 0 1 2 2 2
  spline S106 degree 2 poles (2.9314, -10.4637) (2.9068, -10.3654) (2.8394, -10.2503) (2.7987, -10.2246) knots 0 0 0 1 2 2 2
  spline S107 degree 2 poles (2.7987, -10.2246) (2.7625, -10.2003) (2.6976, -10.1915) (2.6631, -10.2002) knots 0 0 0 1 2 2 2
  spline S108 degree 2 poles (2.6631, -10.2002) (2.5829, -10.2204) (2.5166, -10.359) (2.5439, -10.4675) knots 0 0 0 1 2 2 2
  spline S109 degree 2 poles (2.5439, -10.4675) (2.5593, -10.5288) (2.6106, -10.6003) (2.6523, -10.6199) knots 0 0 0 1 2 2 2
  spline S110 degree 2 poles (2.6523, -10.6199) (2.6826, -10.634) (2.7481, -10.6317) (2.7842, -10.6227) knots 0 0 0 1 2 2 2
  spline S111 degree 2 poles (2.7842, -10.6227) (2.8259, -10.6122) (2.9145, -10.559) (2.9445, -10.5256) knots 0 0 0 1 2 2 2
  spline S112 degree 2 poles (2.9445, -10.5256) (2.9429, -10.516) (2.9364, -10.4833) (2.9314, -10.4637) knots 0 0 0 1 2 2 2
  line L208 (7.9999, -8.2) -> (7.6592, -8.5492)
  line L209 (7.6592, -8.5492) -> (7.5862, -8.4779)
  line L210 (7.5862, -8.4779) -> (7.7129, -8.348)
  line L211 (7.7129, -8.348) -> (7.2333, -7.8799)
  line L212 (7.2333, -7.8799) -> (7.1065, -8.0098)
  line L213 (7.1065, -8.0098) -> (7.041, -7.9459)
  spline S113 degree 2 poles (7.041, -7.9459) (7.1129, -7.8722) (7.139, -7.7618) (7.0855, -7.7006) knots 0 0 0 1 2 2 2
  line L214 (7.0855, -7.7006) -> (7.158, -7.6264)
  line L215 (7.158, -7.6264) -> (7.8029, -8.2557)
  line L216 (7.8029, -8.2557) -> (7.9269, -8.1287)
  line L217 (7.9269, -8.1287) -> (7.9999, -8.2)
  spline S114 degree 2 poles (8.2053, -7.2738) (8.3978, -7.4617) (8.4689, -7.7496) (8.3552, -7.8662) knots 0 0 0 1 2 2 2
  spline S115 degree 2 poles (8.3552, -7.8662) (8.2397, -7.9845) (7.9478, -7.9159) (7.7593, -7.7319) knots 0 0 0 1 2 2 2
  spline S116 degree 2 poles (7.7593, -7.7319) (7.5656, -7.5429) (7.4956, -7.2561) (7.6099, -7.1389) knots 0 0 0 1 2 2 2
  spline S117 degree 2 poles (7.6099, -7.1389) (7.7248, -7.0212) (8.0185, -7.0915) (8.2053, -7.2738) knots 0 0 0 1 2 2 2
  spline S118 degree 2 poles (8.3033, -7.6095) (8.2815, -7.5611) (8.1838, -7.4431) (8.1102, -7.3712) knots 0 0 0 1 2 2 2
  spline S119 degree 2 poles (8.1102, -7.3712) (8.0365, -7.2993) (7.9167, -7.2051) (7.866, -7.1839) knots 0 0 0 1 2 2 2
  spline S120 degree 2 poles (7.866, -7.1839) (7.8154, -7.1628) (7.7284, -7.1764) (7.6894, -7.2164) knots 0 0 0 1 2 2 2
  spline S121 degree 2 poles (7.6894, -7.2164) (7.6503, -7.2565) (7.6376, -7.3449) (7.6606, -7.3967) knots 0 0 0 1 2 2 2
  spline S122 degree 2 poles (7.6606, -7.3967) (7.683, -7.4469) (7.7842, -7.566) (7.8544, -7.6345) knots 0 0 0 1 2 2 2
  spline S123 degree 2 poles (7.8544, -7.6345) (7.9298, -7.7081) (8.0397, -7.7973) (8.0939, -7.8207) knots 0 0 0 1 2 2 2
  spline S124 degree 2 poles (8.0939, -7.8207) (8.1446, -7.843) (8.235, -7.8304) (8.2757, -7.7886) knots 0 0 0 1 2 2 2
  spline S125 degree 2 poles (8.2757, -7.7886) (8.3142, -7.7492) (8.3269, -7.6608) (8.3033, -7.6095) knots 0 0 0 1 2 2 2
  point P0 (0, 0)
  dimension "d129" = 285
  dimension "d133" = 315
  constraints: 212 end point, 2 parallel, 1 horizontal, 1 perpendicular, 196 other
emboss "Emboss1" sketch "Sketch12" operation add depth 0.2 direction (0, 0, -1)
body "Solid1"
